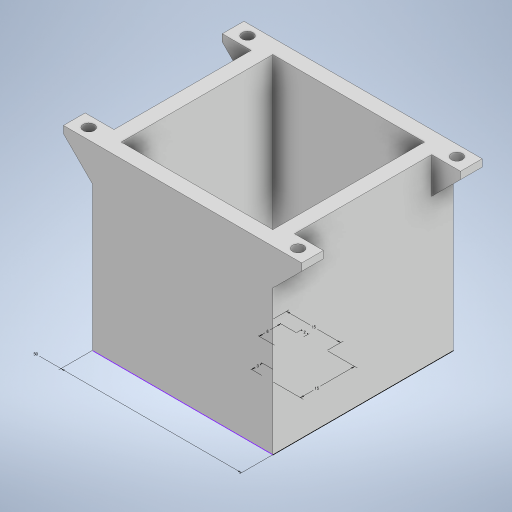
# Autodesk Inventor part: 001_base
Saved by Autodesk Inventor 2024 (Build 280153000, 153)
## iProperties
Created: 2023-11-13
Part Number: 001_base
Material: 一般
Document SubType Name: Modeling
Designer: enmas
Density: 1 g/cm^3
Appearance: 既定
Author: enmas
Autodesk Inventor part; units mm, degrees
ref_plane "YZ Plane" through (0, 0, 0) normal (1, 0, 0) x (0, 1, 0)
ref_plane "XZ Plane" through (0, 0, 0) normal (0, 1, 0) x (-1, 0, 0)
ref_plane "XY Plane" through (0, 0, 0) normal (0, 0, 1) x (1, 0, 0)
sketch "スケッチ1" plane through (0, 0, 0) normal (0, 1, 0) x (-1, 0, 0)
  line L0 (-25, 25) -> (25, 25)
  line L1 (25, 25) -> (25, -25)
  line L2 (25, -25) -> (-25, -25)
  line L3 (-25, -25) -> (-25, 25)
  line L4 (-25, 25) -> (25, -25) construction
  line L5 (25, 25) -> (-25, -25) construction
  line L6 (-7.5, 7.5) -> (7.5, 7.5) construction
  line L7 (7.5, 7.5) -> (7.5, -7.5) construction
  line L8 (7.5, -7.5) -> (-7.5, -7.5) construction
  line L9 (-7.5, -7.5) -> (-7.5, 7.5) construction
  line L10 (-7.5, 7.5) -> (7.5, -7.5) construction
  line L11 (7.5, 7.5) -> (-7.5, -7.5) construction
  line L12 (-7.5, 7.5) -> (-4.5, 7.5)
  line L13 (-4.5, 7.5) -> (-4.5, 4.5)
  line L14 (-4.5, 4.5) -> (-7.5, 4.5)
  line L15 (-7.5, 4.5) -> (-7.5, 7.5)
  line L16 (0, 25) -> (0, -25)
  line L17 (7.5, 7.5) -> (4.5, 7.5)
  line L18 (4.5, 7.5) -> (4.5, 4.5)
  line L19 (4.5, 4.5) -> (7.5, 4.5)
  line L20 (7.5, 4.5) -> (7.5, 7.5)
  line L21 (-1, -1.5) -> (1, -1.5)
  line L22 (1, -1.5) -> (1, -7.5)
  line L23 (1, -7.5) -> (-1, -7.5)
  line L24 (-1, -7.5) -> (-1, -1.5)
  line L25 (-1, -1.5) -> (1, -7.5) construction
  line L26 (1, -1.5) -> (-1, -7.5) construction
  point P0 (0, 0)
  point P1 (0, -4.5)
  dimension "d0" = 50
  dimension "d1" = 15
  dimension "d2" = 15
  dimension "d3" = 3
  dimension "d4" = 2
  dimension "d5" = 6
  constraints: 54 end point, 8 midpoint, 8 parallel, 4 horizontal, 4 perpendicular, 3 point on line, 3 symmetric about line
  measures "d0" distance of L0.start L0.end
  measures "d1" distance of L7.end L8.end
  measures "d2" distance of L8.end L6.start
  measures "d3" distance of L12.end L13.end
  measures "d4" distance of L22.end L23.end
  measures "d5" distance between parallel lines of L23 L21
extrude "押し出し1" add sketch "スケッチ1" along normal blind 4 contours L0 L16 L21 L24 L23 L2 L3 | L0 L1 L2 L16 L23 L22 L21
sketch "スケッチ2" plane through (0, 4, 0) normal (0, 1, 0) x (1, 0, 0)
  line L0 (25, -25) -> (25, 25) projected
  line L1 (25, 25) -> (-25, 25) projected
  line L2 (-25, 25) -> (-25, -25) projected
  line L3 (-25, -25) -> (25, -25) projected
  line L4 (1, 1.5) -> (-1, 1.5) projected
  line L5 (-1, 1.5) -> (-1, 7.5) projected
  line L6 (-1, 7.5) -> (1, 7.5) projected
  line L7 (1, 7.5) -> (1, 1.5) projected
  line L8 (7.5, -7.5) -> (4.5, -7.5) projected
  line L9 (4.5, -7.5) -> (4.5, -4.5) projected
  line L10 (4.5, -4.5) -> (7.5, -4.5) projected
  line L11 (7.5, -4.5) -> (7.5, -7.5) projected
  line L12 (-4.5, -4.5) -> (-4.5, -7.5) projected
  line L13 (-4.5, -7.5) -> (-7.5, -7.5) projected
  line L14 (-7.5, -7.5) -> (-7.5, -4.5) projected
  line L15 (-7.5, -4.5) -> (-4.5, -4.5) projected
  line L16 (-21, 21) -> (21, 21)
  line L17 (21, 21) -> (21, -21)
  line L18 (21, -21) -> (-21, -21)
  line L19 (-21, -21) -> (-21, 21)
  point P0 (0, 0)
  dimension "d8" = 4
  constraints: 8 end point, 3 other
  measures "d8" distance between parallel lines of L1 L16
extrude "押し出し2" add sketch "スケッチ2" along normal blind 46 contours L3 L2 L1 L0
sketch "スケッチ3" plane through (0, 0, 0) normal (0, -1, 0) x (1, 0, 0)
  line L0 (8.2926, -13.4937) -> (21.2256, -13.4937) construction
  line L1 (21.2256, -13.4937) -> (21.2256, -16.6701) construction
  line L2 (21.2256, -16.6701) -> (8.2926, -16.6701) construction
  line L3 (8.2926, -16.6701) -> (8.2926, -13.4937) construction
  spline S0 degree 2 poles (9.7919, -16.6602) (9.4955, -16.6602) (8.9941, -16.4602) (8.8113, -16.2601) knots 0 0 0 1 2 2 2
  spline S1 degree 2 poles (8.8113, -16.2601) (8.6285, -16.0625) (8.4284, -15.4697) (8.4284, -15.0844) knots 0 0 0 1 2 2 2
  spline S2 degree 2 poles (8.4284, -15.0844) (8.4284, -14.7015) (8.6236, -14.1334) (8.8088, -13.9235) knots 0 0 0 1 2 2 2
  spline S3 degree 2 poles (8.8088, -13.9235) (8.9916, -13.7185) (9.4905, -13.5036) (9.7993, -13.5036) knots 0 0 0 1 2 2 2
  spline S4 degree 2 poles (9.7993, -13.5036) (9.9524, -13.5036) (10.2217, -13.548) (10.3353, -13.5826) knots 0 0 0 1 2 2 2
  spline S5 degree 2 poles (10.3353, -13.5826) (10.4341, -13.6147) (10.6391, -13.7061) (10.7404, -13.7604) knots 0 0 0 1 2 2 2
  line L4 (10.7404, -13.7604) -> (10.7404, -14.2495)
  line L5 (10.7404, -14.2495) -> (10.7083, -14.2495)
  spline S6 degree 2 poles (10.7083, -14.2495) (10.6539, -14.2001) (10.486, -14.0618) (10.3649, -13.9951) knots 0 0 0 1 2 2 2
  spline S7 degree 2 poles (10.3649, -13.9951) (10.2488, -13.9309) (9.9747, -13.8494) (9.7968, -13.8494) knots 0 0 0 1 2 2 2
  spline S8 degree 2 poles (9.7968, -13.8494) (9.6017, -13.8494) (9.2534, -14.0099) (9.1225, -14.1631) knots 0 0 0 1 2 2 2
  spline S9 degree 2 poles (9.1225, -14.1631) (8.9941, -14.3187) (8.8508, -14.7904) (8.8508, -15.0844) knots 0 0 0 1 2 2 2
  spline S10 degree 2 poles (8.8508, -15.0844) (8.8508, -15.3981) (9.0015, -15.8501) (9.1324, -16.0057) knots 0 0 0 1 2 2 2
  spline S11 degree 2 poles (9.1324, -16.0057) (9.2608, -16.1564) (9.6042, -16.3095) (9.7968, -16.3095) knots 0 0 0 1 2 2 2
  spline S12 degree 2 poles (9.7968, -16.3095) (9.9722, -16.3095) (10.2711, -16.2231) (10.3872, -16.1588) knots 0 0 0 1 2 2 2
  spline S13 degree 2 poles (10.3872, -16.1588) (10.4983, -16.0946) (10.6638, -15.9612) (10.7107, -15.9143) knots 0 0 0 1 2 2 2
  line L6 (10.7107, -15.9143) -> (10.7404, -15.9143)
  line L7 (10.7404, -15.9143) -> (10.7404, -16.3984)
  spline S14 degree 2 poles (10.7404, -16.3984) (10.6391, -16.4454) (10.4613, -16.5318) (10.3353, -16.5713) knots 0 0 0 1 2 2 2
  spline S15 degree 2 poles (10.3353, -16.5713) (10.2019, -16.6158) (9.9747, -16.6602) (9.7919, -16.6602) knots 0 0 0 1 2 2 2
  line L8 (13.4771, -16.6059) -> (12.951, -16.6059)
  line L9 (12.951, -16.6059) -> (11.9877, -15.3931)
  line L10 (11.9877, -15.3931) -> (11.5234, -15.3931)
  line L11 (11.5234, -15.3931) -> (11.5234, -16.6059)
  line L12 (11.5234, -16.6059) -> (11.1183, -16.6059)
  line L13 (11.1183, -16.6059) -> (11.1183, -13.5579)
  line L14 (11.1183, -13.5579) -> (11.9037, -13.5579)
  spline S16 degree 2 poles (11.9037, -13.5579) (12.1656, -13.5579) (12.5188, -13.6147) (12.6793, -13.7185) knots 0 0 0 1 2 2 2
  spline S17 degree 2 poles (12.6793, -13.7185) (12.8399, -13.8222) (13.0251, -14.1458) (13.0251, -14.3854) knots 0 0 0 1 2 2 2
  spline S18 degree 2 poles (13.0251, -14.3854) (13.0251, -14.7188) (12.6843, -15.1708) (12.3928, -15.2795) knots 0 0 0 1 2 2 2
  line L15 (12.3928, -15.2795) -> (13.4771, -16.6059)
  spline S19 degree 2 poles (12.6028, -14.4175) (12.6028, -14.2841) (12.5089, -14.0791) (12.4101, -14.0124) knots 0 0 0 1 2 2 2
  spline S20 degree 2 poles (12.4101, -14.0124) (12.3236, -13.9556) (12.0939, -13.9086) (11.926, -13.9086) knots 0 0 0 1 2 2 2
  line L16 (11.926, -13.9086) -> (11.5234, -13.9086)
  line L17 (11.5234, -13.9086) -> (11.5234, -15.0547)
  line L18 (11.5234, -15.0547) -> (11.879, -15.0547)
  spline S21 degree 2 poles (11.879, -15.0547) (12.0544, -15.0547) (12.3335, -14.993) (12.4299, -14.8967) knots 0 0 0 1 2 2 2
  spline S22 degree 2 poles (12.4299, -14.8967) (12.5188, -14.8127) (12.6028, -14.5756) (12.6028, -14.4175) knots 0 0 0 1 2 2 2
  spline S23 degree 2 poles (15.8755, -13.9062) (16.0484, -14.1087) (16.2411, -14.7015) (16.2411, -15.0819) knots 0 0 0 1 2 2 2
  spline S24 degree 2 poles (16.2411, -15.0819) (16.2411, -15.4524) (16.0534, -16.0526) (15.8755, -16.2552) knots 0 0 0 1 2 2 2
  spline S25 degree 2 poles (15.8755, -16.2552) (15.6878, -16.4676) (15.1913, -16.6701) (14.8925, -16.6701) knots 0 0 0 1 2 2 2
  spline S26 degree 2 poles (14.8925, -16.6701) (14.5837, -16.6701) (14.0897, -16.4602) (13.9094, -16.2552) knots 0 0 0 1 2 2 2
  spline S27 degree 2 poles (13.9094, -16.2552) (13.734, -16.0526) (13.5463, -15.4573) (13.5463, -15.0819) knots 0 0 0 1 2 2 2
  spline S28 degree 2 poles (13.5463, -15.0819) (13.5463, -14.6991) (13.7365, -14.1161) (13.9119, -13.9062) knots 0 0 0 1 2 2 2
  spline S29 degree 2 poles (13.9119, -13.9062) (14.0897, -13.7036) (14.5862, -13.4937) (14.8925, -13.4937) knots 0 0 0 1 2 2 2
  spline S30 degree 2 poles (14.8925, -13.4937) (15.2037, -13.4937) (15.7026, -13.711) (15.8755, -13.9062) knots 0 0 0 1 2 2 2
  spline S31 degree 2 poles (15.8187, -15.0819) (15.8187, -14.7806) (15.6878, -14.3137) (15.5692, -14.1606) knots 0 0 0 1 2 2 2
  spline S32 degree 2 poles (15.5692, -14.1606) (15.4482, -14.0025) (15.1074, -13.8444) (14.8949, -13.8444) knots 0 0 0 1 2 2 2
  spline S33 degree 2 poles (14.8949, -13.8444) (14.6751, -13.8444) (14.3441, -13.9976) (14.2181, -14.1606) knots 0 0 0 1 2 2 2
  spline S34 degree 2 poles (14.2181, -14.1606) (14.0971, -14.3162) (13.9687, -14.7855) (13.9687, -15.0819) knots 0 0 0 1 2 2 2
  spline S35 degree 2 poles (13.9687, -15.0819) (13.9687, -15.6821) (14.4726, -16.3194) (14.8949, -16.3194) knots 0 0 0 1 2 2 2
  spline S36 degree 2 poles (14.8949, -16.3194) (15.3173, -16.3194) (15.8187, -15.6821) (15.8187, -15.0819) knots 0 0 0 1 2 2 2
  line L19 (16.3572, -16.6059) -> (17.3847, -13.5579)
  line L20 (17.3847, -13.5579) -> (17.8837, -13.5579)
  line L21 (17.8837, -13.5579) -> (18.9112, -16.6059)
  line L22 (18.9112, -16.6059) -> (18.4839, -16.6059)
  line L23 (18.4839, -16.6059) -> (18.2072, -15.7537)
  line L24 (18.2072, -15.7537) -> (17.0438, -15.7537)
  line L25 (17.0438, -15.7537) -> (16.7672, -16.6059)
  line L26 (16.7672, -16.6059) -> (16.3572, -16.6059)
  line L27 (18.0961, -15.4079) -> (17.6243, -13.9729)
  line L28 (17.6243, -13.9729) -> (17.155, -15.4079)
  line L29 (17.155, -15.4079) -> (18.0961, -15.4079)
  spline S37 degree 2 poles (20.0499, -16.6602) (19.7189, -16.6602) (19.2545, -16.5219) (19.0495, -16.4231) knots 0 0 0 1 2 2 2
  line L30 (19.0495, -16.4231) -> (19.0495, -15.9143)
  line L31 (19.0495, -15.9143) -> (19.0791, -15.9143)
  spline S38 degree 2 poles (19.0791, -15.9143) (19.2792, -16.102) (19.7856, -16.3095) (20.0202, -16.3095) knots 0 0 0 1 2 2 2
  spline S39 degree 2 poles (20.0202, -16.3095) (20.3561, -16.3095) (20.6995, -16.0304) (20.6995, -15.8007) knots 0 0 0 1 2 2 2
  spline S40 degree 2 poles (20.6995, -15.8007) (20.6995, -15.6179) (20.5192, -15.3907) (20.324, -15.3338) knots 0 0 0 1 2 2 2
  spline S41 degree 2 poles (20.324, -15.3338) (20.1832, -15.2943) (19.9486, -15.24) (19.7732, -15.1955) knots 0 0 0 1 2 2 2
  spline S42 degree 2 poles (19.7732, -15.1955) (19.6151, -15.1535) (19.3657, -15.0276) (19.2693, -14.9263) knots 0 0 0 1 2 2 2
  spline S43 degree 2 poles (19.2693, -14.9263) (19.1755, -14.825) (19.0717, -14.5533) (19.0717, -14.3755) knots 0 0 0 1 2 2 2
  spline S44 degree 2 poles (19.0717, -14.3755) (19.0717, -14.005) (19.6497, -13.5036) (20.0968, -13.5036) knots 0 0 0 1 2 2 2
  spline S45 degree 2 poles (20.0968, -13.5036) (20.3537, -13.5036) (20.8082, -13.6048) (21.0033, -13.7012) knots 0 0 0 1 2 2 2
  line L32 (21.0033, -13.7012) -> (21.0033, -14.1853)
  line L33 (21.0033, -14.1853) -> (20.9736, -14.1853)
  spline S46 degree 2 poles (20.9736, -14.1853) (20.8279, -14.0519) (20.3734, -13.8543) (20.124, -13.8543) knots 0 0 0 1 2 2 2
  spline S47 degree 2 poles (20.124, -13.8543) (19.8424, -13.8543) (19.4941, -14.1186) (19.4941, -14.3335) knots 0 0 0 1 2 2 2
  spline S48 degree 2 poles (19.4941, -14.3335) (19.4941, -14.5262) (19.6991, -14.7559) (19.8918, -14.8077) knots 0 0 0 1 2 2 2
  spline S49 degree 2 poles (19.8918, -14.8077) (20.0202, -14.8423) (20.3932, -14.9312) (20.5167, -14.9683) knots 0 0 0 1 2 2 2
  spline S50 degree 2 poles (20.5167, -14.9683) (20.8304, -15.0646) (21.1218, -15.4524) (21.1218, -15.7365) knots 0 0 0 1 2 2 2
  spline S51 degree 2 poles (21.1218, -15.7365) (21.1218, -15.9168) (20.9761, -16.2626) (20.8452, -16.3836) knots 0 0 0 1 2 2 2
  spline S52 degree 2 poles (20.8452, -16.3836) (20.6995, -16.517) (20.329, -16.6602) (20.0499, -16.6602) knots 0 0 0 1 2 2 2
  line L34 (10.0735, -21.6244) -> (8.3938, -21.6244)
  line L35 (8.3938, -21.6244) -> (8.3938, -21.3378)
  line L36 (8.3938, -21.3378) -> (9.5893, -19.6533)
  line L37 (9.5893, -19.6533) -> (8.4432, -19.6533)
  line L38 (8.4432, -19.6533) -> (8.4432, -19.3371)
  line L39 (8.4432, -19.3371) -> (10.0512, -19.3371)
  line L40 (10.0512, -19.3371) -> (10.0512, -19.6113)
  line L41 (10.0512, -19.6113) -> (8.8508, -21.3008)
  line L42 (8.8508, -21.3008) -> (10.0735, -21.3008)
  line L43 (10.0735, -21.3008) -> (10.0735, -21.6244)
  spline S53 degree 2 poles (11.427, -21.6762) (10.8787, -21.6762) (10.276, -21.0612) (10.276, -20.4931) knots 0 0 0 1 2 2 2
  spline S54 degree 2 poles (10.276, -20.4931) (10.276, -19.9349) (10.8614, -19.2729) (11.3332, -19.2729) knots 0 0 0 1 2 2 2
  spline S55 degree 2 poles (11.3332, -19.2729) (11.5456, -19.2729) (11.8741, -19.3964) (11.9951, -19.5273) knots 0 0 0 1 2 2 2
  spline S56 degree 2 poles (11.9951, -19.5273) (12.1186, -19.6582) (12.2495, -20.0361) (12.2495, -20.3103) knots 0 0 0 1 2 2 2
  line L44 (12.2495, -20.3103) -> (12.2495, -20.5203)
  line L45 (12.2495, -20.5203) -> (10.6663, -20.5203)
  spline S57 degree 2 poles (10.6663, -20.5203) (10.6663, -20.9179) (11.0664, -21.3403) (11.4221, -21.3403) knots 0 0 0 1 2 2 2
  spline S58 degree 2 poles (11.4221, -21.3403) (11.5481, -21.3403) (11.7926, -21.2835) (11.8914, -21.239) knots 0 0 0 1 2 2 2
  spline S59 degree 2 poles (11.8914, -21.239) (11.9951, -21.1896) (12.1384, -21.1032) (12.1853, -21.0637) knots 0 0 0 1 2 2 2
  line L46 (12.1853, -21.0637) -> (12.2076, -21.0637)
  line L47 (12.2076, -21.0637) -> (12.2076, -21.4836)
  spline S60 degree 2 poles (12.2076, -21.4836) (12.1409, -21.5107) (11.9383, -21.5898) (11.8593, -21.612) knots 0 0 0 1 2 2 2
  spline S61 degree 2 poles (11.8593, -21.612) (11.7481, -21.6441) (11.5654, -21.6762) (11.427, -21.6762) knots 0 0 0 1 2 2 2
  spline S62 degree 2 poles (11.8741, -20.2263) (11.8692, -20.0707) (11.8049, -19.8435) (11.7432, -19.7669) knots 0 0 0 1 2 2 2
  spline S63 degree 2 poles (11.7432, -19.7669) (11.6765, -19.6805) (11.4665, -19.5891) (11.3109, -19.5891) knots 0 0 0 1 2 2 2
  spline S64 degree 2 poles (11.3109, -19.5891) (11.1578, -19.5891) (10.9429, -19.6805) (10.854, -19.7694) knots 0 0 0 1 2 2 2
  spline S65 degree 2 poles (10.854, -19.7694) (10.7675, -19.8608) (10.6786, -20.0806) (10.6663, -20.2263) knots 0 0 0 1 2 2 2
  line L48 (10.6663, -20.2263) -> (11.8741, -20.2263)
  line L49 (13.8526, -19.7496) -> (13.8328, -19.7496)
  spline S66 degree 2 poles (13.8328, -19.7496) (13.7884, -19.7373) (13.692, -19.7323) (13.6253, -19.7323) knots 0 0 0 1 2 2 2
  spline S67 degree 2 poles (13.6253, -19.7323) (13.4697, -19.7323) (13.1635, -19.8682) (13.0251, -20.0016) knots 0 0 0 1 2 2 2
  line L50 (13.0251, -20.0016) -> (13.0251, -21.6244)
  line L51 (13.0251, -21.6244) -> (12.6398, -21.6244)
  line L52 (12.6398, -21.6244) -> (12.6398, -19.3371)
  line L53 (12.6398, -19.3371) -> (13.0251, -19.3371)
  line L54 (13.0251, -19.3371) -> (13.0251, -19.678)
  spline S68 degree 2 poles (13.0251, -19.678) (13.2351, -19.4903) (13.5488, -19.3371) (13.697, -19.3371) knots 0 0 0 1 2 2 2
  spline S69 degree 2 poles (13.697, -19.3371) (13.7563, -19.3371) (13.8155, -19.3421) (13.8526, -19.3495) knots 0 0 0 1 2 2 2
  line L55 (13.8526, -19.3495) -> (13.8526, -19.7496)
  spline S70 degree 2 poles (16.0311, -20.4807) (16.0311, -21.0587) (15.4754, -21.6886) (15.011, -21.6886) knots 0 0 0 1 2 2 2
  spline S71 degree 2 poles (15.011, -21.6886) (14.5343, -21.6886) (13.9884, -21.039) (13.9884, -20.4807) knots 0 0 0 1 2 2 2
  spline S72 degree 2 poles (13.9884, -20.4807) (13.9884, -19.9077) (14.5516, -19.2729) (15.011, -19.2729) knots 0 0 0 1 2 2 2
  spline S73 degree 2 poles (15.011, -19.2729) (15.4754, -19.2729) (16.0311, -19.9052) (16.0311, -20.4807) knots 0 0 0 1 2 2 2
  spline S74 degree 2 poles (15.6335, -20.4807) (15.6335, -20.0361) (15.3099, -19.6039) (15.011, -19.6039) knots 0 0 0 1 2 2 2
  spline S75 degree 2 poles (15.011, -19.6039) (14.7122, -19.6039) (14.3861, -20.0361) (14.3861, -20.4807) knots 0 0 0 1 2 2 2
  spline S76 degree 2 poles (14.3861, -20.4807) (14.3861, -20.913) (14.7122, -21.3576) (15.011, -21.3576) knots 0 0 0 1 2 2 2
  spline S77 degree 2 poles (15.011, -21.3576) (15.3074, -21.3576) (15.6335, -20.9204) (15.6335, -20.4807) knots 0 0 0 1 2 2 2
  point P0 (0, 0)
  constraints: 2 other
extrude "押し出し3" cut sketch "スケッチ3" against normal blind 0.5
sketch "スケッチ4" plane through (0, 50, 0) normal (0, 1, 0) x (1, 0, 0)
  line L0 (25, -25) -> (25, 25) projected
  line L1 (25, 25) -> (33, 25)
  line L2 (33, 25) -> (33, 19)
  line L3 (33, 19) -> (25, 19)
  line L4 (25, 19) -> (25, 25)
  point P0 (0, 0)
  dimension "d13" = 8
  dimension "d14" = 6
  constraints: 8 end point, 2 parallel, 1 horizontal, 1 perpendicular
  measures "d13" distance of L0.end L1.end
  measures "d14" distance of L1.end L2.end
extrude "押し出し4" add sketch "スケッチ4" against normal blind 2
mirror "ミラー1" about plane through (0, 0, 0) normal (1, 0, 0) of "押し出し4"
mirror "ミラー2" about plane through (0, 0, 0) normal (0, 0, 1) of "押し出し4", "ミラー1"
chamfer "面取り2" distance 8 angle 45 4 edges at (25, 48, 22) (25, 48, -22) (-25, 48, -22) (-25, 48, 22)
sketch "スケッチ5" plane through (0, 50, 0) normal (0, 1, 0) x (1, 0, 0)
  line L0 (33, -19) -> (33, -25) projected
  point P0 (0, 0)
  point P1 (29, -22)
  point P2 (29, 22)
  point P3 (-29, 22)
  point P4 (-29, -22)
  dimension "d23" = 4
  measures "d23" distance from line of point (29, -22) L0
hole "穴1" at (29, 50, 22) at (29, 50, -22) at (-29, 50, -22) at (-29, 50, 22) direction (0, -1, 0) diameter 3.1 depth 8 tip angle 118
sketch "スケッチ6" plane through (0, 0, 0) normal (0, -1, 0) x (1, 0, 0)
  line L0 (-4.5, 4.5) -> (-4.5, 7.5) projected
  line L1 (-7.5, 4.5) -> (-4.5, 4.5) projected
  line L2 (-7.5, 7.5) -> (-7.5, 4.5) projected
  line L3 (-4.5, 7.5) -> (-7.5, 7.5) projected
  line L4 (7.5, 7.5) -> (4.5, 7.5) projected
  line L5 (7.5, 4.5) -> (7.5, 7.5) projected
  line L6 (4.5, 4.5) -> (7.5, 4.5) projected
  line L7 (4.5, 7.5) -> (4.5, 4.5) projected
  line L8 (1, -1.5) -> (-1, -1.5) projected
  line L9 (1, -7.5) -> (1, -1.5) projected
  line L10 (-1, -7.5) -> (1, -7.5) projected
  line L11 (-1, -1.5) -> (-1, -7.5) projected
  line L12 (25, 25) -> (25, -25) projected
  line L13 (-25, 25) -> (25, 25) projected
  line L14 (-25, -25) -> (-25, 25) projected
  line L15 (25, -25) -> (-25, -25) projected
  line L16 (13.8526, -19.3495) -> (13.8526, -19.7496) projected
  line L17 (13.8526, -19.7496) -> (13.8328, -19.7496) projected
  line L18 (13.0251, -20.0016) -> (13.0251, -21.6244) projected
  line L19 (13.0251, -21.6244) -> (12.6398, -21.6244) projected
  line L20 (12.6398, -21.6244) -> (12.6398, -19.3371) projected
  line L21 (12.6398, -19.3371) -> (13.0251, -19.3371) projected
  line L22 (13.0251, -19.3371) -> (13.0251, -19.678) projected
  line L23 (12.2495, -20.3103) -> (12.2495, -20.5203) projected
  line L24 (12.2495, -20.5203) -> (10.6663, -20.5203) projected
  line L25 (12.1853, -21.0637) -> (12.2076, -21.0637) projected
  line L26 (12.2076, -21.0637) -> (12.2076, -21.4836) projected
  line L27 (19.0495, -16.4231) -> (19.0495, -15.9143) projected
  line L28 (19.0495, -15.9143) -> (19.0791, -15.9143) projected
  line L29 (21.0033, -13.7012) -> (21.0033, -14.1853) projected
  line L30 (21.0033, -14.1853) -> (20.9736, -14.1853) projected
  line L31 (16.7672, -16.6059) -> (16.3572, -16.6059) projected
  line L32 (16.3572, -16.6059) -> (17.3847, -13.5579) projected
  line L33 (17.3847, -13.5579) -> (17.8837, -13.5579) projected
  line L34 (17.8837, -13.5579) -> (18.9112, -16.6059) projected
  line L35 (18.9112, -16.6059) -> (18.4839, -16.6059) projected
  line L36 (18.4839, -16.6059) -> (18.2072, -15.7537) projected
  line L37 (18.2072, -15.7537) -> (17.0438, -15.7537) projected
  line L38 (17.0438, -15.7537) -> (16.7672, -16.6059) projected
  line L39 (12.3928, -15.2795) -> (13.4771, -16.6059) projected
  line L40 (13.4771, -16.6059) -> (12.951, -16.6059) projected
  line L41 (12.951, -16.6059) -> (11.9877, -15.3931) projected
  line L42 (11.9877, -15.3931) -> (11.5234, -15.3931) projected
  line L43 (11.5234, -15.3931) -> (11.5234, -16.6059) projected
  line L44 (11.5234, -16.6059) -> (11.1183, -16.6059) projected
  line L45 (11.1183, -16.6059) -> (11.1183, -13.5579) projected
  line L46 (11.1183, -13.5579) -> (11.9037, -13.5579) projected
  line L47 (10.7404, -13.7604) -> (10.7404, -14.2495) projected
  line L48 (10.7404, -14.2495) -> (10.7083, -14.2495) projected
  line L49 (10.7107, -15.9143) -> (10.7404, -15.9143) projected
  line L50 (10.7404, -15.9143) -> (10.7404, -16.3984) projected
  line L51 (10.0735, -21.3008) -> (10.0735, -21.6244) projected
  line L52 (10.0735, -21.6244) -> (8.3938, -21.6244) projected
  line L53 (8.3938, -21.6244) -> (8.3938, -21.3378) projected
  line L54 (8.3938, -21.3378) -> (9.5893, -19.6533) projected
  line L55 (9.5893, -19.6533) -> (8.4432, -19.6533) projected
  line L56 (8.4432, -19.6533) -> (8.4432, -19.3371) projected
  line L57 (8.4432, -19.3371) -> (10.0512, -19.3371) projected
  line L58 (10.0512, -19.3371) -> (10.0512, -19.6113) projected
  line L59 (10.0512, -19.6113) -> (8.8508, -21.3008) projected
  line L60 (8.8508, -21.3008) -> (10.0735, -21.3008) projected
  line L61 (-7.5, 7.5) -> (7.5, 7.5)
  line L62 (7.5, 7.5) -> (7.5, -7.5)
  line L63 (7.5, -7.5) -> (-7.5, -7.5)
  line L64 (-7.5, -7.5) -> (-7.5, 7.5)
  point P0 (0, 0)
  point P1 (13.6253, -19.7323)
  point P2 (13.697, -19.3371)
  point P3 (11.8593, -21.612)
  point P4 (11.427, -21.6762)
  point P5 (10.276, -20.4931)
  point P6 (11.3332, -19.2729)
  point P7 (11.9951, -19.5273)
  point P8 (11.4221, -21.3403)
  point P9 (11.8914, -21.239)
  point P10 (20.8452, -16.3836)
  point P11 (20.0499, -16.6602)
  point P12 (20.0202, -16.3095)
  point P13 (20.6995, -15.8007)
  point P14 (20.324, -15.3338)
  point P15 (19.7732, -15.1955)
  point P16 (19.2693, -14.9263)
  point P17 (19.0717, -14.3755)
  point P18 (20.0968, -13.5036)
  point P19 (20.124, -13.8543)
  point P20 (19.4941, -14.3335)
  point P21 (19.8918, -14.8077)
  point P22 (20.5167, -14.9683)
  point P23 (21.1218, -15.7365)
  point P24 (14.8925, -13.4937)
  point P25 (15.8755, -13.9062)
  point P26 (16.2411, -15.0819)
  point P27 (15.8755, -16.2552)
  point P28 (14.8925, -16.6701)
  point P29 (13.9094, -16.2552)
  point P30 (13.5463, -15.0819)
  point P31 (13.9119, -13.9062)
  point P32 (12.6793, -13.7185)
  point P33 (13.0251, -14.3854)
  point P34 (10.3353, -16.5713)
  point P35 (9.7919, -16.6602)
  point P36 (8.8113, -16.2601)
  point P37 (8.4284, -15.0844)
  point P38 (8.8088, -13.9235)
  point P39 (9.7993, -13.5036)
  point P40 (10.3353, -13.5826)
  point P41 (10.3649, -13.9951)
  point P42 (9.7968, -13.8494)
  point P43 (9.1225, -14.1631)
  point P44 (8.8508, -15.0844)
  point P45 (9.1324, -16.0057)
  point P46 (9.7968, -16.3095)
  point P47 (10.3872, -16.1588)
  point P48 (15.011, -19.2729)
  point P49 (16.0311, -20.4807)
  point P50 (15.011, -21.6886)
  point P51 (13.9884, -20.4807)
  point P52 (-11, 0)
  point P53 (11, 0)
  dimension "d31" = 3.5
  dimension "d32" = 3.5
  constraints: 8 end point, 2 parallel, 1 horizontal, 1 perpendicular, 60 other
  measures "d31" distance from line of point (-11, 0) L64
  measures "d32" distance from line of L62 point (11, 0)
hole "穴2" at (-11, 0, 0) at (11, 0, 0) direction (0, 1, 0) diameter 2.1 depth 8 tip angle 118 clearance for "Countersunk Flat Head Screw" size "M2" standard "JIS"
